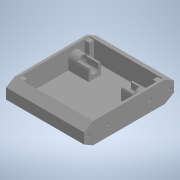
# Autodesk Inventor part: HexBody
Saved by Autodesk Inventor 2020 (Build 240168000, 168)
## iProperties
Created: 2023-12-19
Part Number: HexBody
Material: H TPU
Document SubType Name: Modeling
Designer: smz3rm
Density: 0.941117 g/cm^3
Appearance: Generic(1)
Mass: 193.14 g
Surface Area: 753.57 cm^2
Volume: 205.224 cm^3
BaseThickness: 3.000 mm
TopThickness: 1.778 mm
SideThickness: 4.000 mm
BodyWidth: 130.000 mm
BodyLength: 150.000 mm
BodyHeight: 35.000 mm
DriveMotorHeight: 17.500 mm
WheelWidth: 13.000 mm
WheelGrooveWidth: 4.000 mm
WheelGrooveDia: 15.400 mm
WheelDia: 38.500 mm
WheelPulleyDia: 2.000 mm
M3ScrewInsertBrim: 8.000 mm
M3ScrewDia: 3.100 mm
M3ScrewHeadDia: 6.100 mm
M3ScrewInsertDia: 4.000 mm
M3ScrewInsertDepth: 7.000 mm
DriveMotorOffset: 40.000 mm
DriveMotorHoleDia: 4.200 mm
M3ScrewHeadDepth: 2.200 mm
M3ScrewHeadTaper: -32.50 deg
WheeGuardlSlotWidth: 20.000 mm
WheelGuardScrewOffset: 7.000 mm
FlipperLength: 70.000 mm
FlipperThickness: 4.000 mm
FlipperWidth: 20.000 mm
WheelSpokes: 5.000 ul
FlipperTubeDia: 2.000 mm
Author: smz3rm
Autodesk Inventor part; units mm, degrees
ref_plane "YZ Plane" through (0, 0, 0) normal (1, 0, 0) x (0, 1, 0)
ref_plane "XZ Plane" through (0, 0, 0) normal (0, 1, 0) x (-1, 0, 0)
ref_plane "XY Plane" through (0, 0, 0) normal (0, 0, 1) x (1, 0, 0)
sketch "Sketch1" plane through (0, 0, 0) normal (1, 0, 0) x (0, 1, 0)
  line L0 (-17.5, 75) -> (17.5, 75)
  line L1 (17.5, 75) -> (17.5, -75)
  line L2 (17.5, -75) -> (-17.5, -75)
  line L3 (-17.5, -75) -> (-17.5, 75)
  line L4 (-17.5, 75) -> (17.5, -75) construction
  line L5 (17.5, 75) -> (-17.5, -75) construction
  line L6 (-24.5, 0) -> (24.5, 0) projected
  line L7 (0, -105) -> (0, 105) projected
  line L8 (8.75, -75) -> (-8.75, -75)
  line L9 (-8.75, -75) -> (-17.5, -59.8446)
  line L10 (-17.5, -59.8446) -> (-8.75, -44.6891)
  line L11 (-8.75, -44.6891) -> (8.75, -44.6891)
  line L12 (8.75, -44.6891) -> (17.5, -59.8446)
  line L13 (17.5, -59.8446) -> (8.75, -75)
  line L14 (-8.75, 75) -> (-17.5, 59.8446)
  line L15 (17.5, 59.8446) -> (8.75, 75)
  point P0 (0, 0)
  point P1 (0, -59.8446)
  dimension "d0" = 35
  dimension "d1" = 150
  dimension "d25" = 15.1554
  constraints: 28 end point, 4 point on line, 4 symmetric about line, 2 midpoint, 2 parallel, 1 horizontal, 1 perpendicular, 13 other
  measures "d0" distance of L1.end L2.end
  measures "d1" distance of L0.end L1.end
  measures "d25" distance from line of point (0, -59.845) L2
extrude "Extrusion1" add sketch "Sketch1" along normal mid plane 130 contours L0 L7 L6 L3 L14 | L0 L15 L1 L6 L7 | L6 L7 L11 L10 L3 | L6 L1 L12 L11 L7 | L10 L11 L7 L2 L9 | L11 L12 L13 L2 L7
sketch "Sketch2" plane through (-65, 17.5, 60.2776) normal (0, 1, 0) x (1, 0, 0)
  line L0 (130, 120.1221) -> (130, 0.433) projected
  line L1 (0, 0.433) -> (0, 120.1221) projected
  line L2 (126, 120.1221) -> (4, 120.1221)
  line L3 (4, 120.1221) -> (4, 0.433)
  line L4 (4, 0.433) -> (126, 0.433)
  line L5 (126, 0.433) -> (126, 120.1221)
  line L6 (126, 120.1221) -> (4, 0.433) construction
  line L7 (4, 120.1221) -> (126, 0.433) construction
  line L8 (0, 0.433) -> (130, 0.433) projected
  line L9 (0, 120.1221) -> (130, 120.1221) projected
  point P0 (65, 60.2776)
  dimension "d4" = 4
  constraints: 12 end point, 2 midpoint, 2 parallel, 1 horizontal, 1 perpendicular, 1 point on line
  measures "d4" distance between parallel lines of L1 L3
extrude "Extrusion2" cut sketch "Sketch2" against normal blind 32 contours L5 L4 L3 L2
sketch "Sketch3" plane through (-65, -14.5, 60.2776) normal (0, 1, 0) x (1, 0, 0)
  line L0 (4, 0.433) -> (4, 120.1221) projected
  line L1 (126, 0.433) -> (4, 0.433) projected
  line L2 (126, 120.1221) -> (126, 0.433) projected
  line L3 (4, 120.1221) -> (126, 120.1221) projected
  line L4 (4, 0.433) -> (4, 120.1221) projected
  line L5 (126, 120.1221) -> (126, 0.433) projected
  line L6 (130, 120.1221) -> (130, 0.433) projected
  line L7 (0, 0.433) -> (0, 120.1221) projected
  line L8 (4, 120.1221) -> (12, 120.1221)
  line L9 (12, 120.1221) -> (12, 112.1221)
  line L10 (12, 112.1221) -> (4, 112.1221)
  line L11 (4, 112.1221) -> (4, 120.1221)
  line L12 (-26, 60.2776) -> (156, 60.2776) projected
  line L13 (65, 165.2776) -> (65, -44.7224) projected
  line L14 (118, 120.1221) -> (118, 112.1221)
  line L15 (118, 112.1221) -> (126, 112.1221)
  line L16 (12, 0.433) -> (12, 8.433)
  line L17 (12, 8.433) -> (4, 8.433)
  line L18 (118, 0.433) -> (118, 8.433)
  line L19 (118, 8.433) -> (126, 8.433)
  line L20 (0, 120.1221) -> (4, 120.1221) projected
  line L21 (0, 0.433) -> (4, 0.433) projected
  line L22 (126, 0.433) -> (130, 0.433) projected
  line L23 (126, 120.1221) -> (130, 120.1221) projected
  point P0 (65, 60.2776)
  point P1 (12, 0.433)
  point P2 (4, 112.1221)
  point P3 (126, 8.433)
  point P4 (118, 0.433)
  dimension "d8" = 8
  constraints: 20 end point, 9 symmetric about line, 2 parallel, 2 perpendicular, 1 horizontal
  measures "d8" distance of L9.end L10.end
extrude "Extrusion3" add sketch "Sketch3" along normal blind 30.222 contours L0 L17 L16 L1 | L0 L3 L9 L10 | L18 L19 L2 L1 | L15 L14 L3 L2
sketch "Sketch4" plane through (-61, 17.5, 59.8446) normal (1, 0, 0) x (0, 0, -1)
  circle A0 centre (94.8446, -17.5) radius 8.25
  line L0 (119.6891, -35) -> (0, -35) projected
  line L1 (134.8446, -8.75) -> (134.8446, -26.25) projected
  circle A1 centre (94.8446, -17.5) radius 10.25
  line L2 (84.5946, -17.5) -> (84.5946, -32)
  line L3 (8, -32) -> (111.6891, -32) projected
  line L4 (105.0946, -17.5) -> (105.0946, -32)
  point P0 (59.8446, -17.5)
  dimension "d12" = 16.5
  dimension "d13" = 17.5
  dimension "d14" = 40
  dimension "d15" = 2
  constraints: 4 end point, 2 centre point, 2 point on circle, 2 point on line, 2 tangent, 2 vertical, 1 coincident
  measures "d12" diameter of A0
  measures "d13" distance from line of L0 A0.centre
  measures "d14" distance from line of L1 A0.centre
  measures "d15" radial gap between concentric circles of A0 A1
extrude "Extrusion4" add sketch "Sketch4" along normal blind 14
sketch "Sketch5" plane through (-47, 17.5, 59.8446) normal (1, 0, 0) x (0, 0, -1)
  circle A0 centre (94.8446, -17.5) radius 8.25 projected
  circle A1 centre (94.8446, -17.5) radius 7.75
  line L0 (105.0946, -32) -> (105.0946, -17.5) projected
  arc A2 (105.0946, -17.5) -> (84.5946, -17.5) centre (94.8446, -17.5) ccw projected
  line L1 (84.5946, -17.5) -> (84.5946, -32) projected
  line L2 (105.0946, -32) -> (84.5946, -32) projected
  circle A3 centre (94.8446, -17.5) radius 8.25 projected
  line L3 (88.7446, -12.7196) -> (85.7776, -12.7196)
  arc A4 (105.0946, -17.5) -> (84.5946, -17.5) centre (94.8446, -17.5) ccw projected
  line L4 (88.7446, -12.7196) -> (88.7446, -32)
  line L5 (105.0946, -32) -> (84.5946, -32) projected
  line L6 (100.9446, -12.7196) -> (103.9115, -12.7196)
  line L7 (100.9446, -12.7196) -> (100.9446, -32)
  point P0 (59.8446, -17.5)
  point P1 (88.7446, -22.2804)
  point P2 (85.7776, -12.7196)
  point P3 (100.9446, -22.2804)
  dimension "d18" = 15.5
  dimension "d19" = 12.2
  constraints: 8 end point, 4 point on circle, 2 horizontal, 2 perpendicular, 2 point on line, 1 centre point, 1 coincident, 1 parallel
  measures "d18" diameter of A1
  measures "d19" distance between parallel lines of L7 L4
extrude "Extrusion5" add sketch "Sketch5" along normal blind 20 contours A0 L7 A1 L6 | A0 L6 A2 L0 L2 L7 | L7 L2 L4 A0 | A0 L4 A1 L7 | L3 A1 L4 A0 | A0 L4 L2 L1 A2 L3 | A1 L7 | L4 A1
sketch "Sketch6" plane through (-61, 0, -35) normal (1, 0, 0) x (0, 0, -1)
  circle A0 centre (0, 0) radius 2.1
  point P0 (-35, 0)
  dimension "d22" = 4.2
  constraints: 1 centre point
  measures "d22" diameter of A0
extrude "Extrusion6" cut sketch "Sketch6" against normal through all
mirror "Mirror1" about plane through (0, 0, 0) normal (1, 0, 0) of "Extrusion4", "Extrusion5", "Extrusion6"
sketch "Sketch7" plane through (-65, 0, 0) normal (-1, 0, 0) x (0, 0, 1)
  line L0 (-105, 0) -> (105, 0) projected
  circle A0 centre (35, 0) radius 2
  line L1 (75, -8.75) -> (75, 8.75) projected
  point P0 (0, 0)
  dimension "d26" = 4
  dimension "d27" = 40
  constraints: 1 centre point, 1 point on line
  measures "d26" diameter of A0
  measures "d27" distance from line of L1 A0.centre
extrude "Extrusion7" cut sketch "Sketch7" against normal up to surface (4 mm away)
mirror "Mirror2" about plane through (0, 0, 0) normal (1, 0, 0) of "Extrusion7"
sketch "Sketch9" plane through (-65, 0, 0) normal (-1, 0, 0) x (0, 0, 1)
  line L0 (-59.8446, 17.5) -> (-59.8446, 15.722) projected
  line L1 (-59.8446, -17.5) -> (-59.8446, 17.5)
  line L2 (-75, -8.75) -> (-75, 8.75) projected
  line L3 (-75, 0) -> (-59.8446, 0)
  line L4 (-59.8446, -14.5) -> (-59.8446, 15.722) projected
  circle A0 centre (-67.4223, 0) radius 2
  line L5 (0, -24.5) -> (0, 24.5) projected
  circle A1 centre (67.4223, 0) radius 2
  point P0 (0, 0)
  dimension "d30" = 4
  constraints: 4 end point, 2 centre point, 2 midpoint, 1 perpendicular, 1 point on line, 1 symmetric about line, 1 vertical, 1 other
  measures "d30" diameter of A0
extrude "Extrusion8" cut sketch "Sketch9" against normal blind 7
mirror "Mirror3" about plane through (0, 0, 0) normal (1, 0, 0) of "Extrusion8"
equation "\"d0\" = BodyHeight"
equation "\"d1\" = BodyLength"
equation "\"d2\" = BodyWidth"
equation "\"d4\" = SideThickness"
equation "\"d5\" = BodyHeight - BaseThickness"
equation "\"d8\" = M3ScrewInsertBrim"
equation "\"d10\" = -BaseThickness + BodyHeight - TopThickness"
equation "\"d13\" = DriveMotorHeight"
equation "\"d14\" = DriveMotorOffset"
equation "\"d22\" = DriveMotorHoleDia"
equation "\"d26\" = M3ScrewInsertDia"
equation "\"d27\" = DriveMotorOffset"
equation "\"d30\" = M3ScrewInsertDia"
equation "\"d31\" = M3ScrewInsertDepth"
equation "\"BaseThickness\" = 3"
equation "\"TopThickness\" = 1.778"
equation "\"SideThickness\" = 4"
equation "\"BodyWidth\" = 130"
equation "\"BodyLength\" = 150"
equation "\"BodyHeight\" = 35"
equation "\"DriveMotorHeight\" = 0.5 * BodyHeight"
equation "\"WheelWidth\" = 13"
equation "\"WheelGrooveWidth\" = 4"
equation "\"WheelGrooveDia\" = 0.4 * WheelDia"
equation "\"WheelPulleyDia\" = 2"
equation "\"M3ScrewInsertBrim\" = 8"
equation "\"M3ScrewDia\" = 3.1"
equation "\"M3ScrewHeadDia\" = 6.1"
equation "\"M3ScrewInsertDia\" = 4"
equation "\"M3ScrewInsertDepth\" = 7"
equation "\"DriveMotorOffset\" = 40"
equation "\"DriveMotorHoleDia\" = 4.2"
equation "\"M3ScrewHeadDepth\" = 2.2"
equation "\"M3ScrewHeadTaper\" = -32.5deg"
equation "\"WheelGuardScrewOffset\" = 7"
equation "\"FlipperLength\" = 70"
equation "\"FlipperThickness\" = 4"
equation "\"FlipperWidth\" = 20"
equation "\"WheelSpokes\" = 5"
equation "\"FlipperTubeDia\" = 2"
equation "\"WheelDia\" = 38.5"
body "Solid1"
